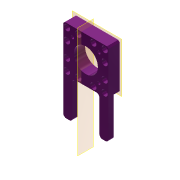
# Autodesk Inventor part: cellSTORM_UC2_Sample_arm
Saved by Autodesk Inventor 2019.4 (Build 234330000, 330)
## iProperties
Created: 2020-12-29
Part Number: cellSTORM_UC2_Sample_arm
Material: Generic
Document SubType Name: Modeling
Designer: diederichbenedict
Density: 1 g/cm^3
Appearance: Smooth - Purple
Author: diederichbenedict
Autodesk Inventor part; units mm, degrees
ref_plane "YZ Plane" through (0, 0, 0) normal (1, 0, 0) x (0, 1, 0)
ref_plane "XZ Plane" through (0, 0, 0) normal (0, 1, 0) x (-1, 0, 0)
ref_plane "XY Plane" through (0, 0, 0) normal (0, 0, 1) x (1, 0, 0)
ref_plane "Work Plane1" through (0, 0, 0) normal (0, 0, 1) x (1, 0, 0)
sketch "Sketch1" plane through (0, 0, 0) normal (0, 0, 1) x (1, 0, 0)
  circle A0 centre (-10, -25) radius 1.45 projected
  circle A1 centre (-10, 25) radius 1.45 projected
  circle A2 centre (10, 25) radius 1.45 projected
  circle A3 centre (10, -25) radius 1.45 projected
  circle A4 centre (-25, 25) radius 2.325 projected
  circle A5 centre (25, -25) radius 2.325 projected
  circle A6 centre (-25, -25) radius 2.325 projected
  circle A7 centre (25, 25) radius 2.325 projected
  line L0 (28, 30) -> (30, 28) projected
  line L1 (28, 30) -> (-28, 30) projected
  line L2 (-30, 28) -> (-28, 30) projected
  line L3 (-30, 28) -> (-30, -28) projected
  line L4 (-28, -30) -> (-30, -28) projected
  line L5 (-28, -30) -> (28, -30) projected
  line L6 (30, -28) -> (28, -30) projected
  line L7 (30, -28) -> (30, 28) projected
  circle A8 centre (-17.5, -17.5) radius 1.95 projected
  circle A9 centre (17.5, 17.5) radius 1.95 projected
  circle A10 centre (17.5, -17.5) radius 1.95 projected
  circle A11 centre (-17.5, 17.5) radius 1.95 projected
  circle A12 centre (0, 0) radius 7.5 projected
  circle A13 centre (-25.33, -75.26) radius 6.15 projected
  circle A14 centre (25, -10) radius 1.45 projected
  circle A15 centre (-25, -10) radius 1.45 projected
  circle A16 centre (-25, 10) radius 1.45 projected
  circle A17 centre (25, 10) radius 1.45 projected
  point P0 (0, 0)
extrude "Extrusion1" add sketch "Sketch1" along normal blind 8 contours L0 L7 L6 L5 L4 L3 L2 L1
sketch "Sketch2" plane through (0, 0, 8) normal (0, 0, 1) x (1, 0, 0)
  circle A0 centre (0, 0) radius 7.5 projected
  circle A1 centre (25, 10) radius 1.45 projected
  circle A2 centre (-25, 10) radius 1.45 projected
  circle A3 centre (-25, -10) radius 1.45 projected
  circle A4 centre (25, -10) radius 1.45 projected
  circle A5 centre (10, -25) radius 1.45 projected
  circle A6 centre (10, 25) radius 1.45 projected
  circle A7 centre (-10, 25) radius 1.45 projected
  circle A8 centre (-10, -25) radius 1.45 projected
  line L0 (-28, -30) -> (28, -30) projected
  line L1 (28, -30) -> (30, -28) projected
  line L2 (30, -28) -> (30, 28) projected
  line L3 (30, 28) -> (28, 30) projected
  line L4 (28, 30) -> (-28, 30) projected
  line L5 (30, -28) -> (30, 28) projected
  line L6 (30, -30) -> (18, -30)
  line L7 (18, -30) -> (18, -80)
  line L8 (18, -80) -> (30, -80)
  line L9 (30, -80) -> (30, -30)
  line L10 (30, 28) -> (30, -28) projected
  line L11 (30, -30) -> (30, -28)
  line L12 (30, -28) -> (28, -30)
  line L13 (-28, 30) -> (-30, 28) projected
  line L14 (-30, 28) -> (-30, -28) projected
  line L15 (-30, -28) -> (-28, -30) projected
  line L16 (-30, -30) -> (-18, -30)
  line L17 (-18, -30) -> (-18, -80)
  line L18 (-18, -80) -> (-30, -80)
  line L19 (-30, -80) -> (-30, -30)
  line L20 (-30, -30) -> (-30, -28)
  line L21 (-30, -28) -> (-28, -30)
  line L22 (-28, -30) -> (-30, -30)
  line L23 (28, -30) -> (30, -28) projected
  line L24 (28, -30) -> (30, -30)
  line L25 (30, -30) -> (30, -28)
  line L26 (30, -28) -> (28, -30)
  circle A9 centre (-17.5, 17.5) radius 1.95 projected
  circle A10 centre (-25, 25) radius 2.325 projected
  circle A11 centre (25, 25) radius 2.325 projected
  circle A12 centre (17.5, 17.5) radius 1.95 projected
  circle A13 centre (17.5, -17.5) radius 1.95 projected
  circle A14 centre (25, -25) radius 2.325 projected
  circle A15 centre (-25, -25) radius 2.325 projected
  point P0 (0, 0)
  point P1 (-24.2387, -104)
  dimension "d57" = 12
  dimension "d58" = 50
  dimension "d59" = 12
  constraints: 32 end point, 5 point on line, 4 parallel, 3 collinear, 3 perpendicular, 2 horizontal, 2 vertical
  measures "d57" distance of L8.end L7.end
  measures "d58" distance of L7.end L6.end
  measures "d59" distance of L17.end L18.end
extrude "Extrusion2" add sketch "Sketch2" along normal blind 7
fillet "Fillet1" radius 4 6 edges at (30, -80, 11.5) (18, -80, 11.5) (-18, -80, 11.5) (-30, -80, 11.5) (-18, -30, 11.5) (18, -30, 11.5)
sketch "Sketch6" plane through (0, 0, 15) normal (0, 0, 1) x (1, 0, 0)
  line L0 (30, -76) -> (30, 28) projected
  line L1 (30, 28) -> (28, 30) projected
  line L2 (28, 30) -> (-28, 30) projected
  circle A0 centre (-1.1442, -37.6316) radius 2.45
  circle A1 centre (-1.1442, -37.6316) radius 1.45 construction
  line L3 (-14, -30) -> (14, -30) projected
  line L4 (18, -34) -> (18, -76) projected
  line L5 (22, -80) -> (26, -80) projected
  line L6 (-28, 30) -> (-30, 28) projected
  line L7 (-30, 28) -> (-30, -76) projected
  line L8 (-26, -80) -> (-22, -80) projected
  line L9 (-18, -76) -> (-18, -34) projected
  arc A2 (-30, -76) -> (-26, -80) centre (-26, -76) ccw projected
  arc A3 (-22, -80) -> (-18, -76) centre (-22, -76) ccw projected
  arc A4 (-14, -30) -> (-18, -34) centre (-14, -34) ccw projected
  arc A5 (18, -34) -> (14, -30) centre (14, -34) ccw projected
  arc A6 (18, -76) -> (22, -80) centre (22, -76) ccw projected
  arc A7 (26, -80) -> (30, -76) centre (26, -76) ccw projected
  point P0 (0, 0)
  dimension "d27" = 4.9
  constraints: 1 centre point, 1 coincident
  measures "d27" diameter of A0
extrude "Extrusion6" cut sketch "Sketch6" against normal blind 4 contours A0
ref_plane "Work Plane2" through (-6, -91, 19) normal (1, 0, 0) x (0, 0, -1)
sketch "Sketch7" plane through (0, 0, 15) normal (0, 0, 1) x (1, 0, 0)
  circle A0 centre (10, -25) radius 1.45 projected
  circle A1 centre (-10, -25) radius 1.45 projected
  circle A2 centre (-25, -10) radius 1.45 projected
  circle A3 centre (-25, 10) radius 1.45 projected
  circle A4 centre (-10, 25) radius 1.45 projected
  circle A5 centre (10, 25) radius 1.45 projected
  circle A6 centre (25, 10) radius 1.45 projected
  circle A7 centre (25, -10) radius 1.45 projected
  circle A8 centre (-25, 25) radius 2.325 projected
  circle A9 centre (25, 25) radius 2.325 projected
  circle A10 centre (25, -25) radius 2.325 projected
  circle A11 centre (-25, -25) radius 2.325 projected
  point P0 (0, 0)
hole "Hole1" at (-25, -10, 15) at (-25, 10, 15) at (-10, 25, 15) at (10, 25, 15) at (25, 10, 15) at (25, -10, 15) at (10, -25, 15) at (-10, -25, 15) at (-25, 25, 15) at (-25, -25, 15) at (25, -25, 15) at (25, 25, 15) direction (0, 0, -1) diameter 3.2 end through all counterbore diameter 8 counterbore depth 10
sketch "Sketch8" plane through (0, 0, 15) normal (0, 0, 1) x (1, 0, 0)
  circle A0 centre (0, 0) radius 16
  dimension "d41" = 32
  constraints: 1 centre point, 1 coincident
  measures "d41" diameter of A0
extrude "Extrusion7" cut sketch "Sketch8" against normal through all
chamfer "Chamfer3" distance 5 angle 45 2 edges at (21, -30, 8) (-21, -30, 8)
sketch "Sketch10" plane through (0, 0, 8) normal (0, 0, -1) x (-1, 0, 0)
  line L0 (-23, -35) -> (-30, -28) projected
  line L1 (-30, -76) -> (-30, -28) projected
  arc A0 (-30, -76) -> (-26, -80) centre (-26, -76) ccw projected
  line L2 (-22, -80) -> (-26, -80) projected
  arc A1 (-22, -80) -> (-18, -76) centre (-22, -76) ccw projected
  line L3 (-18, -35) -> (-18, -76) projected
  line L4 (-23, -35) -> (-18, -35) projected
  line L5 (18, -35) -> (23, -35) projected
  line L6 (18, -35) -> (18, -76) projected
  arc A2 (18, -76) -> (22, -80) centre (22, -76) ccw projected
  line L7 (22, -80) -> (26, -80) projected
  arc A3 (26, -80) -> (30, -76) centre (26, -76) ccw projected
  line L8 (30, -28) -> (30, -76) projected
  line L9 (30, -28) -> (23, -35) projected
  circle A4 centre (-24, -70) radius 2.45
  circle A5 centre (24, -70) radius 2.45
  circle A6 centre (-24, -58) radius 2.45
  circle A7 centre (24, -58) radius 2.45
  circle A8 centre (-24, -46) radius 2.45
  circle A9 centre (24, -46) radius 2.45
  point P0 (0, 0)
  dimension "d63" = 4.9
  dimension "d64" = 4.9
  dimension "d65" = 4.9
  dimension "d66" = 4.9
  dimension "d67" = 4.9
  dimension "d68" = 4.9
  dimension "d69" = 10
  dimension "d70" = 12
  dimension "d71" = 12
  dimension "d72" = 10
  dimension "d73" = 12
  dimension "d74" = 12
  constraints: 6 centre point
  measures "d63" diameter of A4
  measures "d64" diameter of A5
  measures "d65" diameter of A6
  measures "d66" diameter of A7
  measures "d67" diameter of A8
  measures "d68" diameter of A9
  measures "d69" distance from line of A4.centre L2
  measures "d70" distance of A6.centre A4.centre
  measures "d71" distance of A8.centre A6.centre
  measures "d72" distance from line of A5.centre L7
  measures "d73" distance of A7.centre A5.centre
  measures "d74" distance of A9.centre A7.centre
extrude "Extrusion9" cut sketch "Sketch10" against normal blind 6 contours A4 | A5 | A6 | A7 | A8 | A9
body "Solid1"
